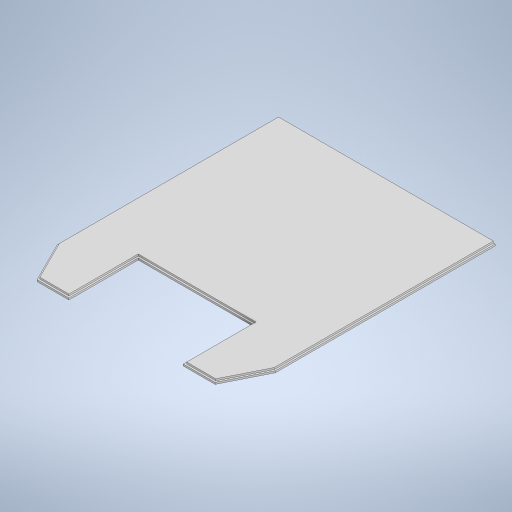
# Autodesk Inventor part: Bot v1 top
Saved by Autodesk Inventor 2024 (Build 280153000, 153)
## iProperties
Created: 2023-10-22
Part Number: Bot v1 top
Material: Generic
Document SubType Name: Modeling
Designer: CJ110
Density: 1 g/cm^3
Appearance: Default
Author: CJ110
Autodesk Inventor part; units mm, degrees
ref_plane "YZ Plane" through (0, 0, 0) normal (1, 0, 0) x (0, 1, 0)
ref_plane "XZ Plane" through (0, 0, 0) normal (0, 1, 0) x (-1, 0, 0)
ref_plane "XY Plane" through (0, 0, 0) normal (0, 0, 1) x (1, 0, 0)
sketch "Sketch1" plane through (0, 0, 0) normal (0, 1, 0) x (-1, 0, 0)
  line L0 (-50.8, 241.3) -> (-50.8, 177.8)
  line L1 (-50.8, 177.8) -> (-152.4, 177.8)
  line L2 (-152.4, 177.8) -> (-152.4, 241.3)
  line L3 (-152.4, 241.3) -> (-184.15, 241.3)
  line L4 (-184.15, 241.3) -> (-203.2, 203.2)
  line L5 (-203.2, 0) -> (-203.2, 203.2)
  line L6 (0, 0) -> (-203.2, 0)
  line L7 (0, 203.2) -> (0, 0)
  line L8 (0, 203.2) -> (-19.05, 241.3)
  line L9 (-19.05, 241.3) -> (-50.8, 241.3)
  dimension "d14" = 177.8
  dimension "d15" = 203.2
  dimension "d16" = 63.5
  dimension "d17" = 38.1
  dimension "d18" = 50.8
  dimension "d19" = 31.75
  constraints: 20 end point, 4 equal length, 4 perpendicular, 2 parallel, 1 coincident, 1 collinear, 1 vertical
  measures "d14" distance between parallel lines of L1 L6
  measures "d15" distance between parallel lines of L5 L7
  measures "d16" distance between parallel lines of L1 L9
  measures "d17" distance from line of L7.start L9
  measures "d18" distance between parallel lines of L0 L7
  measures "d19" distance of L9.start L9.end
extrude "Extrusion1" add sketch "Sketch1" along normal blind 1.5875
sketch "Sketch2" plane through (0, 1.5875, 0) normal (0, 1, 0) x (1, 0, 0)
  line L0 (19.05, -241.3) -> (50.8, -241.3) projected
  line L1 (50.8, -241.3) -> (50.8, -177.8) projected
  line L2 (50.8, -177.8) -> (152.4, -177.8) projected
  line L3 (152.4, -177.8) -> (152.4, -241.3) projected
  line L4 (152.4, -241.3) -> (184.15, -241.3) projected
  line L5 (184.15, -241.3) -> (203.2, -203.2) projected
  line L6 (203.2, -203.2) -> (203.2, 0) projected
  line L7 (203.2, 0) -> (0, 0) projected
  line L8 (0, 0) -> (0, -203.2) projected
  line L9 (0, -203.2) -> (19.05, -241.3) projected
  line L10 (201.6125, -1.5875) -> (201.6125, -202.8252)
  line L11 (201.6125, -202.8252) -> (183.1689, -239.7125)
  line L12 (183.1689, -239.7125) -> (153.9875, -239.7125)
  line L13 (153.9875, -239.7125) -> (153.9875, -176.2125)
  line L14 (153.9875, -176.2125) -> (49.2125, -176.2125)
  line L15 (49.2125, -176.2125) -> (49.2125, -239.7125)
  line L16 (49.2125, -239.7125) -> (20.0311, -239.7125)
  line L17 (20.0311, -239.7125) -> (1.5875, -202.8252)
  line L18 (1.5875, -202.8252) -> (1.5875, -1.5875)
  line L19 (1.5875, -1.5875) -> (201.6125, -1.5875)
  dimension "d22" = 1.5875
  constraints: 20 end point, 9 other
  measures "d22" distance between parallel lines of L6 L10
extrude "Extrusion2" cut sketch "Sketch2" against normal up to next
sketch "Sketch3" plane through (0, 1.5875, 0) normal (0, 1, 0) x (1, 0, 0)
  line L0 (183.1689, -239.7125) -> (201.6125, -202.8252) projected
  line L1 (201.6125, -202.8252) -> (201.6125, -1.5875) projected
  line L2 (201.6125, -1.5875) -> (1.5875, -1.5875) projected
  line L3 (1.5875, -1.5875) -> (1.5875, -202.8252) projected
  line L4 (1.5875, -202.8252) -> (20.0311, -239.7125) projected
  line L5 (20.0311, -239.7125) -> (49.2125, -239.7125) projected
  line L6 (49.2125, -239.7125) -> (49.2125, -176.2125) projected
  line L7 (49.2125, -176.2125) -> (153.9875, -176.2125) projected
  line L8 (153.9875, -176.2125) -> (153.9875, -239.7125) projected
  line L9 (153.9875, -239.7125) -> (183.1689, -239.7125) projected
  line L10 (200.025, -3.175) -> (200.025, -202.4505)
  line L11 (200.025, -202.4505) -> (182.1877, -238.125)
  line L12 (182.1877, -238.125) -> (155.575, -238.125)
  line L13 (155.575, -238.125) -> (155.575, -174.625)
  line L14 (155.575, -174.625) -> (47.625, -174.625)
  line L15 (47.625, -174.625) -> (47.625, -238.125)
  line L16 (47.625, -238.125) -> (21.0123, -238.125)
  line L17 (21.0123, -238.125) -> (3.175, -202.4505)
  line L18 (3.175, -202.4505) -> (3.175, -3.175)
  line L19 (3.175, -3.175) -> (200.025, -3.175)
  line L20 (3.175, -3.175) -> (3.175, -1.5875)
  line L21 (200.025, -3.175) -> (200.025, -1.5875)
  point P0 (0, 0)
  dimension "d25" = 1.5875
  constraints: 24 end point, 2 perpendicular, 2 point on line, 9 other
  measures "d25" distance between parallel lines of L1 L10
extrude "Extrusion3" add sketch "Sketch3" along normal blind 1.5875 contours L21 L19 L20 L2 | L10 L11 L12 L13 L14 L15 L16 L17 L18 L19
body "Solid1"
